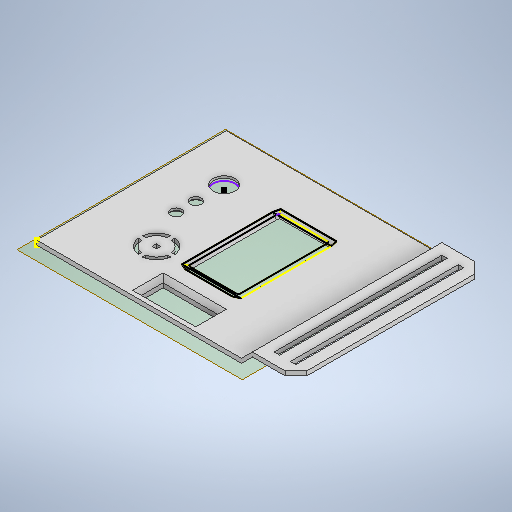
# Autodesk Inventor part: Part2edd
Saved by Autodesk Inventor 2025.2 (Build 292293000, 293)
## iProperties
Created: 2025-06-05
Part Number: Part2edd
Material: Generic
Document SubType Name: Sheet Metal
Designer: ziyuz
Density: 1 g/cm^3
Sheet Metal Rule: Default_mm
Appearance: Default
Author: ziyuz
Autodesk Inventor part; units mm, degrees
ref_plane "YZ Plane" through (0, 0, 0) normal (1, 0, 0) x (0, 1, 0)
ref_plane "XZ Plane" through (0, 0, 0) normal (0, 1, 0) x (-1, 0, 0)
ref_plane "XY Plane" through (0, 0, 0) normal (0, 0, 1) x (1, 0, 0)
sketch "Sketch1" plane through (0, 0, 0) normal (0, 1, 0) x (-1, 0, 0)
  line L0 (0, 0) -> (-94, 0)
  line L1 (-94, 0) -> (-94, -87)
  line L2 (-94, -87) -> (0, -87)
  line L3 (0, -87) -> (0, 0)
  dimension "d0" = 94
  dimension "d1" = 87
  constraints: 8 end point, 2 parallel, 1 horizontal, 1 perpendicular
  measures "d0" distance of L2.end L1.end
  measures "d1" distance of L1.end L0.end
extrude "Extrusion1" add sketch "Sketch1" along normal blind 2
sketch "Sketch2" plane through (0, 0, 0) normal (0, 0, 1) x (1, 0, 0)
  line L0 (94, 2) -> (0, 2) projected
  line L1 (-0.0001, 2) -> (94, 2)
  line L2 (94, 2) -> (99, 7)
  line L3 (94, 2) -> (101.071, 2) construction
  line L4 (94, 0) -> (99, 5)
  line L5 (99, 5) -> (114, 5)
  line L6 (114, 5) -> (114, 7)
  line L7 (114, 7) -> (99, 7)
  line L8 (94, 0) -> (94, 2) projected
  line L9 (94, 0) -> (94, 2)
  point P0 (0, 0)
  dimension "d4" = 7.071
  dimension "d5" = 45
  dimension "d6" = 7.071
  dimension "d7" = 15
  dimension "d8" = 2
  constraints: 16 end point, 3 horizontal, 2 perpendicular, 1 collinear, 1 equal length
  measures "d4" distance of L0.start L2.end
  measures "d5" angle of L3 L2
  measures "d6" distance of L4.start L4.end
  measures "d7" distance of L4.end L5.end
  measures "d8" distance of L5.end L6.end
extrude "Extrusion2" add sketch "Sketch2" against normal blind 87
sketch "Sketch3" plane through (99, 7, 0) normal (0, 1, 0) x (1, 0, 0)
  line L0 (15, 0) -> (0, 0) projected
  line L1 (15, 0) -> (20, 5)
  line L2 (15, 0) -> (22.071, 0) construction
  line L3 (20, 5) -> (20, 82)
  line L4 (0, 87) -> (15, 87) projected
  line L5 (20, 82) -> (15, 87)
  line L6 (15, 0) -> (15, 87)
  point P0 (-99, 0)
  dimension "d11" = 7.071
  dimension "d12" = 45
  dimension "d13" = 77
  constraints: 10 end point, 1 equal length, 1 horizontal, 1 vertical
  measures "d11" distance of L0.start L1.end
  measures "d12" angle of L2 L1
  measures "d13" distance of L1.end L3.end
extrude "Extrusion3" add sketch "Sketch3" against normal blind 2
sketch "Sketch4" plane through (0, 2, 0) normal (0, 1, 0) x (1, 0, 0)
  line L0 (0, 0) -> (94, 0) projected
  line L1 (0, 0) -> (0, 4)
  line L2 (0, 87) -> (0, 0) projected
  line L3 (0, 4) -> (94, 4)
  line L4 (0, 4) -> (44, 4)
  line L5 (44, 4) -> (44, 14)
  line L6 (44, 14) -> (69, 14)
  line L7 (69, 14) -> (69, 4)
  dimension "d16" = 4
  dimension "d17" = 44
  dimension "d18" = 10
  dimension "d19" = 25
  constraints: 12 end point, 4 perpendicular, 3 point on line
  measures "d16" distance of L0.start L1.end
  measures "d17" distance of L1.end L4.end
  measures "d18" distance of L4.end L5.end
  measures "d19" distance of L5.end L6.end
extrude "Extrusion4" cut sketch "Sketch4" against normal blind 10
ref_plane "Work Plane1" through (0, -2, 0) normal (0, -1, 0) x (1, 0, 0)
sketch "Sketch6" plane through (0, -2, 0) normal (0, -1, 0) x (1, 0, 0)
  line L0 (44, -4) -> (44, -14) projected
  line L1 (44, -4) -> (44, -2)
  line L2 (0, 0) -> (94, 0) projected
  line L3 (44, -2) -> (42, -2)
  line L4 (42, -2) -> (71, -2)
  line L5 (71, -2) -> (71, -16)
  line L6 (71, -16) -> (42, -16)
  line L7 (42, -16) -> (42, -2)
  line L8 (44, -4) -> (69, -4) projected
  line L9 (44, -14) -> (69, -14)
  line L10 (69, -14) -> (69, -4)
  line L11 (69, -4) -> (44, -4)
  line L12 (44, -4) -> (44, -14)
  dimension "d23" = 2
  dimension "d24" = 2
  dimension "d25" = 29
  dimension "d26" = 14
  constraints: 20 end point, 4 parallel, 4 perpendicular, 2 horizontal
  measures "d23" distance of L0.start L1.end
  measures "d24" distance of L1.end L3.end
  measures "d25" distance of L5.end L6.end
  measures "d26" distance of L4.end L5.end
extrude "Extrusion5" add sketch "Sketch6" against normal blind 2
chamfer "Chamfer1" distance 2 angle 45 4 edges at (44, 2, -9) (56.5, 2, -14) (69, 2, -9) (56.5, 2, -4)
sketch "Sketch8" plane through (0, 2, 0) normal (0, 1, 0) x (1, 0, 0)
  line L0 (0, 0) -> (0, 25)
  line L1 (0, 87) -> (0, 0) projected
  line L2 (0, 25) -> (30, 25)
  circle A0 centre (30, 25) radius 7.5
  line L3 (30, 17.5) -> (30, 32.5)
  line L4 (37.5, 25) -> (22.5, 25)
  circle A1 centre (30, 25) radius 6
  line L5 (37.5, 25) -> (30, 25)
  line L6 (30, 25) -> (24, 25)
  line L7 (30, 25) -> (33.75, 25)
  line L8 (30, 25) -> (31.875, 25)
  line L9 (30, 25) -> (30.9375, 25)
  line L10 (30.9375, 25) -> (30.9375, 32.4412)
  line L11 (30.9375, 25) -> (28.9715, 25)
  line L12 (28.9715, 25) -> (28.9715, 32.4291)
  line L13 (30.9375, 25) -> (30.9375, 17.5588)
  line L14 (28.9715, 25) -> (28.9715, 17.5709)
  line L15 (30, 25) -> (30, 24.017)
  line L16 (30, 24.017) -> (30, 25.983)
  line L17 (37.4353, 25.983) -> (22.5647, 25.983)
  line L18 (37.4353, 24.017) -> (22.5647, 24.017)
  point P0 (30.9375, 24.017)
  point P1 (30.9375, 25.983)
  point P2 (28.9715, 25.983)
  point P3 (28.9715, 24.017)
  point P4 (24.0811, 25.983)
  point P5 (28.9715, 30.9112)
  point P6 (24.0811, 24.017)
  point P7 (28.9715, 19.0888)
  point P8 (35.9189, 24.017)
  point P9 (30.9375, 19.0737)
  point P10 (35.9189, 25.983)
  point P11 (30.9375, 30.9263)
  dimension "d34" = 15
  dimension "d35" = 12
  dimension "d32" = 25
  dimension "d33" = 30
  dimension "d36" = 1.966
  dimension "d37" = 0.983
  dimension "d38" = 1.966
  constraints: 36 end point, 8 point on line, 7 midpoint, 3 perpendicular, 2 coincident, 1 collinear, 1 horizontal, 1 parallel, 1 vertical, 13 other
  measures "d32" distance of L0.start L0.end
  measures "d33" distance of L0.end L2.end
  measures "d36" distance of L9.end L11.end
  measures "d37" distance of L5.end L15.end
  measures "d38" distance of L15.end L16.end
extrude "Extrusion6" cut sketch "Sketch8" against normal blind 2 contours A0 L12 A1 L17 | L18 A1 L14 A0 | L12 L17 L3 L2 | L2 L3 L18 L14 | L4 L13 L18 L3 | L3 L17 L10 L4 | A0 L17 A1 L10 | L13 A1 L18 A0
sketch "Sketch9" plane through (0, 2, 0) normal (0, 1, 0) x (1, 0, 0)
  line L0 (0, 0) -> (0, 43)
  line L1 (0, 87) -> (0, 0) projected
  line L2 (0, 43) -> (21, 43)
  circle A0 centre (21, 43) radius 2.5
  line L3 (0, 0) -> (0, 52)
  line L4 (0, 52) -> (21, 52)
  circle A1 centre (21, 52) radius 2.5
  line L5 (0, 0) -> (0, 65)
  line L6 (0, 65) -> (21, 65)
  circle A2 centre (21, 65) radius 5
  dimension "d41" = 43
  dimension "d42" = 21
  dimension "d43" = 90
  dimension "d44" = 5
  dimension "d45" = 52
  dimension "d46" = 5
  dimension "d47" = 65
  dimension "d48" = 21
  dimension "d49" = 10
  constraints: 12 end point, 3 centre point, 3 coincident, 3 perpendicular, 3 point on line
  measures "d41" distance of L0.start L0.end
  measures "d42" distance of L0.end L2.end
  measures "d43" angle of L0 L2
  measures "d44" diameter of A0
  measures "d45" distance of L0.start L3.end
  measures "d46" diameter of A1
  measures "d47" distance of L0.start L5.end
  measures "d48" distance of L5.end L6.end
  measures "d49" diameter of A2
extrude "Extrusion7" cut sketch "Sketch9" against normal blind 2
sketch "Sketch10" plane through (0, 2, 0) normal (0, 1, 0) x (1, 0, 0)
  line L0 (0, 87) -> (0, 0) projected
  line L1 (0, 0) -> (43, 0)
  line L2 (0, 0) -> (94, 0) projected
  line L3 (43, 0) -> (43, 45)
  line L4 (71, 2) -> (42, 2) projected
  line L5 (71, 2) -> (70, 2)
  line L6 (70, 2) -> (70, 45)
  line L7 (70, 45) -> (74, 45) construction
  line L8 (70, 45) -> (70, 65)
  line L9 (70, 45) -> (90, 45) construction
  line L10 (70, 65) -> (67.7057, 68.2766)
  line L11 (67.7057, 68.2766) -> (45.2943, 68.2766)
  line L12 (43, 45) -> (43, 65)
  line L13 (43, 65) -> (45.2943, 68.2766)
  line L14 (70, 45) -> (70, 25)
  line L15 (70, 25) -> (66.8775, 22.5)
  line L16 (43, 45) -> (43, 25)
  line L17 (43, 25) -> (46.1225, 22.5)
  line L18 (46.1225, 22.5) -> (66.8775, 22.5)
  line L19 (66.8775, 22.5) -> (66.8775, 24.5)
  line L20 (70, 25) -> (68, 25)
  line L21 (68, 25) -> (66.8775, 24.5)
  line L22 (70, 65) -> (68, 65)
  line L23 (67.7057, 68.2766) -> (67.7057, 66.2766)
  line L24 (45.2943, 68.2766) -> (45.2943, 66.2766)
  line L25 (43, 65) -> (45, 65)
  line L26 (46.1225, 22.5) -> (46.1225, 24.5)
  line L27 (43, 25) -> (45, 25)
  line L28 (45, 25) -> (45, 65)
  line L29 (45, 65) -> (45.2943, 66.2766)
  line L30 (45.2943, 66.2766) -> (67.7057, 66.2766)
  line L31 (67.7057, 66.2766) -> (68, 65)
  line L32 (68, 65) -> (68, 25)
  line L33 (66.8775, 24.5) -> (46.1225, 24.5)
  line L34 (46.1225, 24.5) -> (45, 25)
  dimension "d52" = 43
  dimension "d53" = 45
  dimension "d54" = 1
  dimension "d58" = 20
  dimension "d59" = 90
  dimension "d60" = 20
  dimension "d61" = 4
  dimension "d62" = 20
  dimension "d63" = 4
  dimension "d64" = 2
  dimension "d65" = 2
  dimension "d66" = 2
  dimension "d67" = 2
  dimension "d68" = 2
  dimension "d69" = 2
  dimension "d70" = 2
  dimension "d71" = 2
  constraints: 64 end point, 8 perpendicular, 6 horizontal, 6 vertical, 4 point on line
  measures "d52" distance of L0.end L1.end
  measures "d53" distance of L1.end L3.end
  measures "d54" distance of L4.start L5.end
  measures "d58" distance of L6.end L8.end
  measures "d59" angle of L9 L8
  measures "d60" distance of L6.end L14.end
  measures "d61" distance of L14.end L15.end
  measures "d62" distance of L3.end L16.end
  measures "d63" distance of L16.end L17.end
  measures "d64" distance of L15.end L19.end
  measures "d65" distance of L14.end L20.end
  measures "d66" distance of L8.end L22.end
  measures "d67" distance of L10.end L23.end
  measures "d68" distance of L11.end L24.end
  measures "d69" distance of L12.end L25.end
  measures "d70" distance of L17.end L26.end
  measures "d71" distance of L16.end L27.end
extrude "Extrusion8" cut sketch "Sketch10" against normal blind 2 contours L28 L29 L30 L31 L32 L21 L33 L34
chamfer "Chamfer2" distance 2 angle 45 8 edges at (45, 2, -45) (45.5612, 2, -24.75) (56.5, 2, -24.5) (67.4388, 2, -24.75) (68, 2, -45) (56.5, 2, -66.2766) (45.1472, 2, -65.6383) (67.8528, 2, -65.6383)
sketch "Sketch11" plane through (0, 2, 0) normal (0, 1, 0) x (1, 0, 0)
  line L0 (45.6972, 22.5) -> (67.3028, 22.5) projected
  line L1 (67.3028, 22.5) -> (45.6972, 22.5)
  line L2 (43, 23.7014) -> (45.6972, 22.5) projected
  line L3 (45.6972, 22.5) -> (43, 23.7014)
  line L4 (43, 23.7014) -> (45, 25) projected
  line L5 (43, 65.2276) -> (43, 23.7014) projected
  line L6 (43, 23.7014) -> (43, 65.2276)
  line L7 (43.7029, 68.2766) -> (45.2943, 66.2766) projected
  line L8 (43, 65.2276) -> (43.7029, 68.2766)
  line L9 (70, 23.7014) -> (70, 65.2276) projected
  line L10 (43, 23.7014) -> (70, 23.7014)
  line L11 (70, 65.2276) -> (68, 65) projected
  line L12 (43, 65.2276) -> (70, 65.2276)
  line L13 (69.2971, 68.2766) -> (43.7029, 68.2766) projected
  line L14 (43.7029, 68.2766) -> (69.2971, 68.2766)
  line L15 (45.6972, 22.5) -> (67.3028, 22.5)
  line L16 (43, 65.2276) -> (43.7029, 68.2766)
  line L17 (43.7029, 68.2766) -> (69.2971, 68.2766)
  line L18 (46.1225, 24.5) -> (66.8775, 24.5) projected
  line L19 (66.8775, 24.5) -> (46.1225, 24.5)
  line L20 (45.6972, 22.5) -> (43, 23.7014)
  line L21 (43, 23.7014) -> (43, 65.2276)
  line L22 (43, 65.2276) -> (43.7029, 68.2766)
  line L23 (69.2971, 68.2766) -> (43.7029, 68.2766)
  line L24 (70, 65.2276) -> (69.2971, 68.2766) projected
  line L25 (69.2971, 68.2766) -> (70, 65.2276)
  line L26 (67.3028, 22.5) -> (70, 23.7014) projected
  line L27 (67.3028, 22.5) -> (70, 23.7014)
  line L28 (68, 25) -> (68, 65) projected
  line L29 (66.8775, 24.5) -> (68, 25)
  line L30 (68, 65) -> (68, 25)
  line L31 (66.8775, 24.5) -> (46.1225, 24.5)
  line L32 (45, 25) -> (46.1225, 24.5) projected
  line L33 (46.1225, 24.5) -> (45, 25)
  line L34 (45, 25) -> (45, 65)
  line L35 (45, 65) -> (45.2943, 66.2766)
  line L36 (67.7057, 66.2766) -> (45.2943, 66.2766) projected
  line L37 (68, 65) -> (67.7057, 66.2766)
  point P0 (0, 0)
  constraints: 48 end point, 9 collinear, 3 horizontal, 3 perpendicular, 3 vertical
sketch "Sketch12" plane through (99, 7, 0) normal (0, 1, 0) x (1, 0, 0)
  line L0 (20, 5) -> (15, 0) projected
  line L1 (20, 5) -> (0, 5)
  line L2 (0, 0) -> (0, 87) projected
  line L3 (15, 87) -> (20, 82) projected
  line L4 (20, 82) -> (0, 82)
  line L5 (10, 82) -> (10, 5)
  line L6 (0, 5) -> (10, 5)
  line L7 (5, 5) -> (5, 82)
  line L8 (10, 5) -> (20, 5)
  line L9 (15, 5) -> (15, 82)
  line L10 (10, 5) -> (15, 5)
  line L11 (10, 5) -> (5, 5)
  line L12 (7.5, 5) -> (7.5, 82)
  line L13 (12.5, 82) -> (12.5, 5)
  point P0 (-99, 0)
  point P1 (7.5, 5)
  point P2 (5, 5)
  point P3 (12.5, 5)
  point P4 (15, 5)
  constraints: 22 end point, 6 midpoint, 5 point on line, 4 collinear, 3 perpendicular, 2 horizontal
extrude "Extrusion9" cut sketch "Sketch12" against normal blind 2 contours L1 L13 L4 L9 | L1 L7 L4 L12
sketch "Sketch13" plane through (0, 0, 0) normal (0, -1, 0) x (1, 0, 0)
  circle A0 centre (21, -52) radius 2.5 projected
  circle A1 centre (21, -52) radius 3.5
  circle A2 centre (21, -43) radius 2.5 projected
  circle A3 centre (21, -43) radius 3.5
  circle A4 centre (21, -65) radius 5 projected
  circle A5 centre (21, -65) radius 7.5
  point P0 (0, 0)
  dimension "d79" = 7
  dimension "d80" = 7
  dimension "d81" = 15
  constraints: 3 centre point, 3 coincident
  measures "d79" diameter of A1
  measures "d80" diameter of A3
  measures "d81" diameter of A5
extrude "Extrusion10" cut sketch "Sketch13" against normal blind 1
sketch "Sketch14" plane through (0, 0, 0) normal (0, -1, 0) x (1, 0, 0)
  circle A0 centre (21, -65) radius 5 projected
  circle A1 centre (21, -65) radius 5
  point P0 (0, 0)
  constraints: 1 centre point, 1 coincident
equation "\"BendRadius\" = Thickness"
equation "\"BendReliefWidth\" = Thickness"
equation "\"BendReliefDepth\" = 0.5 * Thickness"
equation "\"CornerReliefSize\" = 4 * Thickness"
equation "\"MinimumRemnant\" = 2 * Thickness"
equation "\"TransitionRadius\" = BendRadius"
equation "\"JacobiRadiusSize\" = BendRadius"
equation "\"GapSize\" = Thickness"
equation "\"Thickness\" = 0.5"
body "Solid1"
